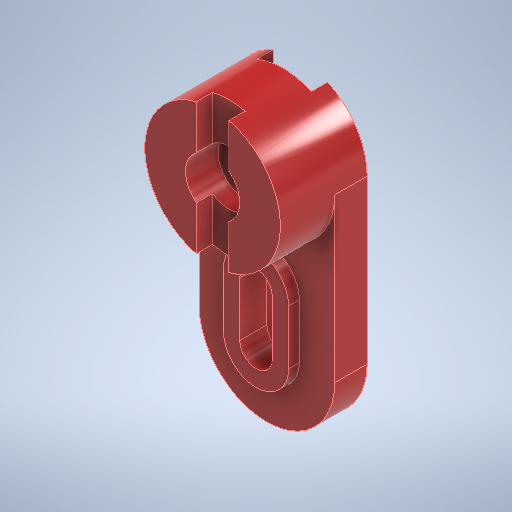
# Autodesk Inventor part: cad@67
Saved by Autodesk Inventor 2025.2 (Build 292293000, 293)
## iProperties
Created: 2025-04-22
Part Number: cad@67
Material: Generic
Document SubType Name: Modeling
Designer: spars
Density: 1 g/cm^3
Appearance: Red
Author: spars
Autodesk Inventor part; units mm, degrees
ref_plane "YZ Plane" through (0, 0, 0) normal (1, 0, 0) x (0, 1, 0)
ref_plane "XZ Plane" through (0, 0, 0) normal (0, 1, 0) x (-1, 0, 0)
ref_plane "XY Plane" through (0, 0, 0) normal (0, 0, 1) x (1, 0, 0)
sketch "Sketch1" plane through (0, 0, 0) normal (0, 0, 1) x (1, 0, 0)
  line L0 (-25, 30) -> (25, 30)
  line L1 (25, 30) -> (25, -30)
  line L2 (25, -30) -> (-25, -30)
  line L3 (-25, -30) -> (-25, 30)
  line L4 (-25, 30) -> (25, -30) construction
  line L5 (25, 30) -> (-25, -30) construction
  arc A0 (-25, -30) -> (25, -30) centre (0, -30) ccw
  point P0 (0, 0)
  dimension "d0" = 50
  dimension "d1" = 60
  dimension "d2" = 25
  constraints: 12 end point, 2 midpoint, 2 parallel, 2 point on circle, 1 centre point, 1 horizontal, 1 perpendicular
  measures "d0" distance of L1.end L2.end
  measures "d1" distance of L0.end L1.end
  measures "d2" radius of A0
extrude "Extrusion1" add sketch "Sketch1" along normal blind 12
sketch "Sketch2" plane through (0, 0, 12) normal (0, 0, 1) x (1, 0, 0)
  line L0 (25, 30) -> (-25, 30) projected
  circle A0 centre (0, 30) radius 25
  point P0 (0, 0)
  dimension "d5" = 50
  constraints: 1 centre point, 1 midpoint
  measures "d5" diameter of A0
extrude "Extrusion2" add sketch "Sketch2" along normal blind 20 and the other way blind 12
sketch "Sketch3" plane through (0, 30, 32) normal (0, 0, 1) x (1, 0, 0)
  line L0 (-6, -25) -> (6, -25)
  line L1 (6, 25) -> (-6, 25)
  line L2 (-6, -25) -> (6, 25) construction
  line L3 (6, -25) -> (-6, 25) construction
  line L4 (-6, 25) -> (-6, 8)
  line L5 (-6, -8) -> (-6, -25)
  line L6 (6, -25) -> (6, -8)
  line L7 (6, 8) -> (6, 25)
  arc A0 (-6, 8) -> (-6, -8) centre (0, 0) ccw
  arc A1 (6, -8) -> (6, 8) centre (0, 0) ccw
  point P0 (0, -30)
  dimension "d11" = 12
  dimension "d12" = 50
  constraints: 16 end point, 5 parallel, 4 point on circle, 2 centre point, 2 midpoint, 2 perpendicular, 1 horizontal
  measures "d11" distance of L1.end L1.start
  measures "d12" distance of L1.start L0.end
extrude "Extrusion3" cut sketch "Sketch3" against normal blind 6
sketch "Sketch4" plane through (0, 30, 26) normal (0, 0, 1) x (1, 0, 0)
  arc A0 (6, -8) -> (6, 8) centre (0, 0) ccw projected
  circle A1 centre (0, 0) radius 10
  point P0 (0, -30)
  point P1 (6, 8)
  point P2 (6, -8)
  dimension "d15" = 20
  constraints: 1 centre point, 1 coincident
  measures "d15" diameter of A1
extrude "Extrusion4" cut sketch "Sketch4" against normal blind 6
sketch "Sketch5" plane through (0, 0, 12) normal (0, 0, 1) x (1, 0, 0)
  arc A0 (-25, -30) -> (25, -30) centre (0, -30) ccw projected
  line L0 (0, -30) -> (0, -10) construction
  line L1 (12, -30) -> (12, -10)
  line L2 (-12, -10) -> (-12, -30)
  arc A1 (-12, -30) -> (12, -30) centre (0, -30) ccw
  arc A2 (12, -10) -> (-12, -10) centre (0, -10) ccw
  line L3 (-6, -10) -> (-6, -30)
  arc A3 (-6, -30) -> (6, -30) centre (0, -30) ccw
  line L4 (6, -30) -> (6, -10)
  arc A4 (6, -10) -> (-6, -10) centre (0, -10) ccw
  point P0 (0, 0)
  point P1 (0, -20)
  dimension "d21" = 12
  dimension "d22" = 6
  constraints: 12 end point, 8 point on circle, 4 centre point, 4 tangent, 2 parallel, 1 midpoint, 1 vertical, 3 other
  measures "d21" radius of A1
  measures "d22" radial gap between concentric circles of A2 A4
extrude "Extrusion5" add sketch "Sketch5" along normal blind 4
sketch "Sketch6" plane through (0, 0, 0) normal (0, 1, 0) x (-1, 0, 0)
  line L0 (-25, 0) -> (25, 0) projected
  line L1 (-10.3999, 0) -> (9.6001, 0)
  line L2 (9.6001, 0) -> (9.6001, 6)
  line L3 (9.6001, 6) -> (-10.3999, 6)
  line L4 (-10.3999, 6) -> (-10.3999, 0)
  point P0 (0, 0)
  point P1 (9.6001, 0)
  dimension "d25" = 20
  dimension "d26" = 6
  constraints: 8 end point, 2 parallel, 1 horizontal, 1 perpendicular
  measures "d25" distance of L3.end L2.end
  measures "d26" distance of L2.end L1.end
extrude "Extrusion6" cut sketch "Sketch6" along normal blind 60 and the other way blind 60
sketch "Sketch7" plane through (0, 0, 12) normal (0, 0, 1) x (1, 0, 0)
  arc A0 (6, -10) -> (-6, -10) centre (0, -10) ccw projected
  line L0 (0, -4) -> (0, -36) construction
  arc A1 (-6, -30) -> (6, -30) centre (0, -30) ccw projected
  line L1 (6, -10) -> (6, -30)
  line L2 (-6, -30) -> (-6, -10)
  arc A2 (6, -10) -> (-6, -10) centre (0, -10) ccw
  arc A3 (-6, -30) -> (6, -30) centre (0, -30) ccw
  point P0 (0, 0)
  point P1 (0, -20)
  constraints: 8 end point, 8 point on circle, 4 tangent, 2 centre point, 2 point on line, 1 midpoint, 1 parallel, 1 vertical
extrude "Extrusion7" cut sketch "Sketch7" against normal through all
body "Solid1"
